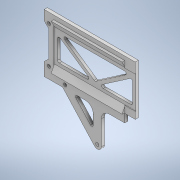
# Autodesk Inventor part: Part1
Saved by Autodesk Inventor 2021 (Build 250183000, 183)
## iProperties
Created: 2025-06-15
Part Number: Part1
Material: Generic
Document SubType Name: Modeling
Designer: Toby
Density: 1 g/cm^3
Appearance: Default
Author: Toby
Autodesk Inventor part; units mm, degrees
ref_plane "YZ Plane" through (0, 0, 0) normal (1, 0, 0) x (0, 1, 0)
ref_plane "XZ Plane" through (0, 0, 0) normal (0, 1, 0) x (-1, 0, 0)
ref_plane "XY Plane" through (0, 0, 0) normal (0, 0, 1) x (1, 0, 0)
sketch "Sketch1" plane through (0, 0, 0) normal (0, 0, 1) x (1, 0, 0)
  line L0 (-26.0453, 15.4617) -> (23.9547, 15.4617)
  line L1 (23.9547, 15.4617) -> (23.9547, -18.5383)
  line L2 (23.9547, -18.5383) -> (-26.0453, -18.5383)
  line L3 (-26.0453, -18.5383) -> (-26.0453, 15.4617)
  point P0 (0, 0)
  dimension "d0" = 50
  dimension "d1" = 34
  constraints: 8 end point, 2 parallel, 1 horizontal, 1 perpendicular
  measures "d0" distance of L0.start L0.end
  measures "d1" distance of L2.end L0.start
extrude "Extrusion1" add sketch "Sketch1" along normal blind 2
sketch "Sketch2" plane through (0, 0, 2) normal (0, 0, 1) x (1, 0, 0)
  line L0 (-26.0453, 15.4617) -> (-26.0453, -18.5383) projected
  line L1 (23.9547, 15.4617) -> (-26.0453, 15.4617) projected
  point P0 (0, 0)
  point P1 (-23.0453, 11.4617)
  point P2 (-23.0453, -11.5383)
  point P3 (-13.0453, -16.5383)
  dimension "d4" = 23
  dimension "d5" = 3
  dimension "d6" = 3
  dimension "d7" = 4
  dimension "d8" = 5
  dimension "d9" = 10
  measures "d4" distance of point (-23.045, -11.538) point (-23.045, 11.462)
  measures "d5" distance from line of L0 point (-23.045, 11.462)
  measures "d6" distance from line of L0 point (-23.045, -11.538)
  measures "d7" distance from line of L1 point (-23.045, 11.462)
  measures "d8" vertical distance of point (-13.045, -16.538) point (-23.045, -11.538)
  measures "d9" horizontal distance of point (-13.045, -16.538) point (-23.045, -11.538)
hole "Hole1" at (-23.0453, 11.4617, 2) at (-23.0453, -11.5383, 2) at (-13.0453, -16.5383, 2) direction (0, 0, -1) diameter 2 depth 6.5 tip angle 118
sketch "Sketch3" plane through (0, 0, 2) normal (0, 0, 1) x (1, 0, 0)
  line L0 (-26.0453, 15.4617) -> (-26.0453, -18.5383) projected
  line L1 (-26.0453, 8.4617) -> (-23.0453, 8.4617)
  line L2 (-23.0453, 8.4617) -> (-23.0453, -7.5383)
  line L3 (-23.0453, -7.5383) -> (-26.0453, -7.5383)
  line L4 (-26.0453, -7.5383) -> (-26.0453, 8.4617)
  line L5 (23.9547, 15.4617) -> (-26.0453, 15.4617) projected
  circle A0 centre (-23.0453, -11.5383) radius 1 projected
  point P0 (0, 0)
  dimension "d17" = 7
  dimension "d18" = 4
  dimension "d19" = 3
  constraints: 8 end point, 2 parallel, 1 horizontal, 1 perpendicular, 1 point on line
  measures "d17" distance between parallel lines of L5 L1
  measures "d18" distance from line of A0.centre L3
  measures "d19" distance between parallel lines of L0 L2
extrude "Extrusion2" cut sketch "Sketch3" against normal blind 2 contours L1 L2 L3 L0
chamfer "Chamfer1" distance 3 angle 45 2 edges at (-26.0453, 8.4617, 1) (-26.0453, -7.5383, 1)
sketch "Sketch5" plane through (0, 0, 2) normal (0, 0, 1) x (1, 0, 0)
  line L0 (-20.0453, 14.9617) -> (23.9547, 14.9617)
  line L1 (23.9547, 14.9617) -> (23.9547, -13.0383)
  line L2 (23.9547, -13.0383) -> (-20.0453, -13.0383)
  line L3 (-20.0453, -13.0383) -> (-20.0453, 14.9617)
  line L4 (23.9547, 15.4617) -> (-26.0453, 15.4617) projected
  line L5 (-26.0453, -18.5383) -> (23.9547, -18.5383) projected
  line L6 (-23.0453, 8.4617) -> (-23.0453, -7.5383) projected
  line L7 (23.9547, -18.5383) -> (23.9547, 15.4617) projected
  circle A0 centre (-13.0453, -16.5383) radius 1 projected
  point P0 (0, 0)
  dimension "d27" = 3
  dimension "d28" = 0
  dimension "d29" = 50
  dimension "d30" = 3.5
  dimension "d31" = 31.5
  dimension "d32" = 0.5
  constraints: 8 end point, 2 parallel, 1 horizontal, 1 perpendicular
  measures "d27" distance between parallel lines of L6 L3
  measures "d28" distance between parallel lines of L7 L1
  measures "d29" distance of L4.start L4.end
  measures "d30" distance from line of A0.centre L2
  measures "d31" distance from line of A0.centre L0
  measures "d32" distance between parallel lines of L4 L0
extrude "Extrusion3" cut sketch "Sketch5" against normal blind 0.4 contours L0 L1 L2 L3
sketch "Sketch8" plane through (0, 0, 2) normal (0, 0, 1) x (1, 0, 0)
  line L0 (-26.0453, -18.5383) -> (23.9547, -18.5383) projected
  line L1 (11.9547, -18.5383) -> (-1.0453, -18.5383)
  line L2 (-1.0453, -18.5383) -> (-1.0453, -44.5383)
  line L3 (-1.0453, -44.5383) -> (11.9547, -44.5383)
  line L4 (11.9547, -44.5383) -> (11.9547, -18.5383)
  line L5 (23.9547, -18.5383) -> (23.9547, 15.4617) projected
  circle A0 centre (-13.0453, -16.5383) radius 1 projected
  line L6 (6.9547, -38.5383) -> (6.9547, -18.5383) construction
  line L7 (9.4547, -38.5383) -> (9.4547, -18.5383)
  line L8 (4.4547, -18.5383) -> (4.4547, -38.5383)
  arc A1 (4.4547, -38.5383) -> (9.4547, -38.5383) centre (6.9547, -38.5383) ccw
  arc A2 (9.4547, -18.5383) -> (4.4547, -18.5383) centre (6.9547, -18.5383) ccw
  circle A3 centre (6.9547, -38.5383) radius 1
  point P0 (0, 0)
  point P1 (23.9547, -13.0383)
  point P2 (6.9547, -28.5383)
  dimension "d48" = 12
  dimension "d49" = 25
  dimension "d50" = 20
  dimension "d51" = 22
  dimension "d52" = 6
  dimension "d53" = 5
  dimension "d54" = 2
  constraints: 16 end point, 4 point on circle, 4 tangent, 3 centre point, 3 parallel, 2 perpendicular, 2 point on line, 1 coincident, 1 horizontal, 1 midpoint
  measures "d48" distance between parallel lines of L5 L4
  measures "d49" distance between parallel lines of L5 L2
  measures "d50" horizontal distance of L6.start A0.centre
  measures "d51" vertical distance of L6.start A0.centre
  measures "d52" distance from line of L3 L6.start
  measures "d53" diameter of A2
  measures "d54" diameter of A3
extrude "Extrusion6" add sketch "Sketch8" against normal blind 2 contours L0 L7 A1 L8
fillet "Fillet1" radius 5 2 edges at (4.4547, -18.5383, 1) (9.4547, -18.5383, 1)
sketch "Sketch9" plane through (0, 0, 2) normal (0, 0, 1) x (1, 0, 0)
  circle A0 centre (-13.0453, -16.5383) radius 1 projected
  circle A1 centre (6.9547, -38.5383) radius 1 projected
  line L0 (-13.0453, -16.5383) -> (6.9547, -38.5383) construction
  line L1 (-14.8951, -18.22) -> (5.1049, -40.22)
  line L2 (8.8046, -36.8566) -> (-11.1954, -14.8566)
  arc A2 (-11.1954, -14.8566) -> (-14.8951, -18.22) centre (-13.0453, -16.5383) ccw
  arc A3 (5.1049, -40.22) -> (8.8046, -36.8566) centre (6.9547, -38.5383) ccw
  line L3 (-26.0453, -18.5383) -> (-0.5453, -18.5383) projected
  line L4 (-14.6058, -18.5383) -> (-7.8485, -18.5383)
  line L5 (4.4547, -23.5383) -> (4.4547, -38.5383) projected
  line L6 (4.4547, -32.0718) -> (4.4547, -38.5383)
  line L7 (4.4547, -38.5383) -> (6.7171, -41.027)
  arc A4 (4.4547, -38.5383) -> (9.4547, -38.5383) centre (6.9547, -38.5383) ccw projected
  point P0 (0, 0)
  point P1 (-3.0453, -27.5383)
  constraints: 14 end point, 6 point on line, 5 point on circle, 4 tangent, 2 centre point, 1 collinear, 1 midpoint, 1 parallel
extrude "Extrusion7" add sketch "Sketch9" against normal blind 2 contours L3 L2 L5 A4 L1
fillet "Fillet2" radius 1 2 edges at (-7.8485, -18.5383, 1) (4.4547, -32.0718, 1)
sketch "Sketch10" plane through (-26.0453, 15.4617, 0) normal (0, 1, 0) x (1, 0, 0)
  line L0 (50, 0) -> (50, -2) projected
  line L1 (0, 0) -> (0, -2) projected
  line L2 (50, -2) -> (0, -2)
  line L3 (0, -2) -> (0, 0)
  line L4 (0, 0) -> (50, 0)
  line L5 (50, 0) -> (50, -2)
  point P0 (26.0453, 0)
  constraints: 8 end point, 2 parallel, 1 horizontal, 1 perpendicular
extrude "Extrusion8" add sketch "Sketch10" along normal blind 2
sketch "Sketch13" plane through (23.9547, -18.5383, 2) normal (1, 0, 0) x (0, 0, -1)
  line L0 (0, 0) -> (0, 5.5) projected
  line L1 (0.4, 5.5) -> (0.4, 33.5) projected
  line L2 (0.4, 5.5) -> (0, 5.5) projected
  line L3 (-1.6, 5.5) -> (0.4, 9.5)
  line L4 (0, 5.5) -> (0.4, 5.5) projected
  line L5 (-1.6, 5.5) -> (0.4, 5.5)
  line L6 (0.4, 5.5) -> (0.4, 9.5)
  point P0 (2, 18.5383)
  point P1 (0.4, 30.4)
  dimension "d70" = 1.6
  dimension "d71" = 4
  constraints: 6 end point, 1 horizontal, 1 perpendicular, 1 point on line
  measures "d70" distance from line of L0 L3.start
  measures "d71" distance from line of L2 L3.end
extrude "Extrusion11" add sketch "Sketch13" against normal blind 44
sketch "Sketch14" plane through (23.9547, -18.5383, 2) normal (1, 0, 0) x (0, 0, -1)
  line L0 (0, 33.5) -> (0, 36) projected
  line L1 (0.4, 33.5) -> (0.4, 9.5) projected
  line L2 (0, 33.5) -> (0.4, 33.5) projected
  line L3 (-1.6, 33.5) -> (0.4, 29.5)
  line L4 (-1.6, 33.5) -> (0.4, 33.5)
  line L5 (0.4, 29.5) -> (0.4, 33.5)
  point P0 (2, 18.5383)
  dimension "d74" = 1.6
  dimension "d75" = 4
  constraints: 6 end point, 1 collinear, 1 perpendicular, 1 point on line
  measures "d74" distance from line of L0 L3.start
  measures "d75" distance from line of L2 L3.end
extrude "Extrusion12" add sketch "Sketch14" against normal blind 44
sketch "Sketch15" plane through (0, 0, 0) normal (0, 0, -1) x (-1, 0, 0)
  line L0 (-23.9547, -18.5383) -> (-23.9547, 17.4617) projected
  line L1 (-23.9547, 17.4617) -> (-30.4547, 17.4617)
  line L2 (-30.4547, 17.4617) -> (-30.4547, -13.3383)
  line L3 (-30.4547, -13.3383) -> (-23.9547, -13.3383)
  line L4 (-23.9547, -13.3383) -> (-23.9547, 17.4617)
  line L5 (-14.4547, -18.5383) -> (-23.9547, -18.5383) projected
  point P0 (0, 0)
  dimension "d78" = 5.2
  dimension "d79" = 6.5
  constraints: 8 end point, 2 parallel, 1 horizontal, 1 perpendicular
  measures "d78" distance between parallel lines of L5 L3
  measures "d79" distance between parallel lines of L0 L2
extrude "Extrusion13" add sketch "Sketch15" against normal blind 2
sketch "Sketch16" plane through (0, 0, 2) normal (0, 0, 1) x (1, 0, 0)
  line L0 (30.4547, -13.3383) -> (30.4547, 17.4617) projected
  line L1 (-20.0453, -9.0383) -> (23.9547, -9.0383) projected
  line L2 (30.4547, 10.9617) -> (-20.0453, 10.9617)
  line L3 (-20.0453, 10.9617) -> (-20.0453, -9.0383)
  line L4 (-20.0453, -9.0383) -> (30.4547, -9.0383)
  line L5 (30.4547, -9.0383) -> (30.4547, 10.9617)
  line L6 (23.9547, 10.9617) -> (-20.0453, 10.9617) projected
  point P0 (0, 0)
  point P1 (30.4547, -9.0383)
  constraints: 8 end point, 2 parallel, 1 collinear, 1 horizontal, 1 perpendicular, 1 point on line
extrude "Extrusion14" cut sketch "Sketch16" against normal blind 0.4
sketch "Sketch17" plane through (0, 0, 1.6) normal (0, 0, 1) x (1, 0, 0)
  line L0 (28.4547, -7.0383) -> (-18.0453, -7.0383)
  line L1 (-18.0453, -7.0383) -> (-18.0453, 8.9617)
  line L2 (-18.0453, 8.9617) -> (28.4547, 8.9617)
  line L3 (28.4547, 8.9617) -> (28.4547, -7.0383)
  line L4 (30.4547, -9.0383) -> (23.9547, -9.0383) projected
  line L5 (23.9547, 10.9617) -> (30.4547, 10.9617) projected
  line L6 (30.4547, 10.9617) -> (30.4547, -9.0383) projected
  line L7 (-20.0453, -9.8383) -> (-20.0453, 11.7617) projected
  point P0 (0, 0)
  dimension "d84" = 2
  dimension "d85" = 2
  dimension "d86" = 2
  dimension "d87" = 2
  constraints: 8 end point, 2 parallel, 1 horizontal, 1 perpendicular
  measures "d84" distance between parallel lines of L0 L4
  measures "d85" distance between parallel lines of L5 L2
  measures "d86" distance between parallel lines of L6 L3
  measures "d87" distance between parallel lines of L7 L1
extrude "Extrusion15" cut sketch "Sketch17" against normal blind 2
sketch "Sketch18" plane through (0, 0, 1.6) normal (0, 0, 1) x (1, 0, 0)
  line L0 (-18.0453, -7.0383) -> (28.4547, -7.0383) projected
  line L1 (28.4547, 8.9617) -> (-18.0453, 8.9617) projected
  line L2 (5.2047, -7.0383) -> (28.4547, 8.9617) construction
  line L3 (5.7716, -7.8621) -> (29.0216, 8.1379)
  line L4 (27.8878, 9.7855) -> (4.6378, -6.2145)
  arc A0 (4.6378, -6.2145) -> (5.7716, -7.8621) centre (5.2047, -7.0383) ccw
  arc A1 (29.0216, 8.1379) -> (27.8878, 9.7855) centre (28.4547, 8.9617) ccw
  line L5 (5.2047, -7.0383) -> (-18.0453, 8.9617) construction
  line L6 (5.7716, -6.2145) -> (-17.4784, 9.7855)
  line L7 (-18.6122, 8.1379) -> (4.6378, -7.8621)
  arc A2 (4.6378, -7.8621) -> (5.7716, -6.2145) centre (5.2047, -7.0383) ccw
  arc A3 (-17.4784, 9.7855) -> (-18.6122, 8.1379) centre (-18.0453, 8.9617) ccw
  point P0 (0, 0)
  point P1 (16.5637, 8.9617)
  point P2 (-8.738, 9.9617)
  point P3 (16.8297, 0.9617)
  point P4 (-6.4203, 0.9617)
  point P5 (4.6378, -7.8621)
  point P6 (5.2047, -5.8244)
  dimension "d90" = 46.5
  dimension "d91" = 2
  dimension "d92" = 2
  constraints: 16 end point, 8 point on circle, 8 tangent, 4 centre point, 3 midpoint, 2 parallel, 1 point on line
  measures "d90" distance of L0.start L0.end
  measures "d91" diameter of A1
  measures "d92" diameter of A3
extrude "Extrusion16" add sketch "Sketch18" against normal blind 1.6 contours L7 A3 L6 L4 A0 L0 | L0 A0 L7 | A0 L4 L6 A2 L0 | L0 A2 A0 | A2 L6 L4 A1 L3 L0 | L0 L3 A2
fillet "Fillet3" radius 1 9 edges at (28.4547, -7.0383, 0.8) (28.4547, 7.7478, 0.8) (26.6907, 8.9617, 0.8) (6.9687, -7.0383, 0.8) (5.2047, -5.8244, 0.8) (3.4407, -7.0383, 0.8) (-16.2813, 8.9617, 0.8) (-18.0453, 7.7478, 0.8) (-18.0453, -7.0383, 0.8)
body "Solid1"
